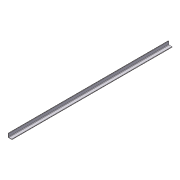
# Autodesk Inventor part: GE-12019-01
Saved by Autodesk Inventor 2012 (Build 160160000, 160)
## iProperties
Created: 2011-06-10
Part Number: GE-12019-01
Document SubType Name: Modeling
Designer: dfoster
Density: 2.71 g/cm^3
Material: Aluminum-6061
Mass: 4666.94 g
Surface Area: 5570.98 cm^2
Volume: 1722.12 cm^3
Description: Angle, Side
Title: Angle, Side
Author: dfoster
Autodesk Inventor part; units mm, degrees
ref_plane "YZ Plane" through (0, 0, 0) normal (1, 0, 0) x (0, 1, 0)
ref_plane "XZ Plane" through (0, 0, 0) normal (0, 1, 0) x (-1, 0, 0)
ref_plane "XY Plane" through (0, 0, 0) normal (0, 0, 1) x (1, 0, 0)
sketch "Sketch1" plane through (0, 0, 0) normal (0, 0, 1) x (1, 0, 0)
  line L0 (0, 0) -> (0, 50.8)
  line L1 (0, 50.8) -> (3.175, 50.8)
  line L2 (50.8, 0) -> (0, 0)
  line L3 (6.35, 47.625) -> (6.35, 12.7)
  line L4 (12.7, 6.35) -> (47.625, 6.35)
  line L5 (50.8, 3.175) -> (50.8, 0)
  arc A0 (6.35, 12.7) -> (12.7, 6.35) centre (12.7, 12.7) ccw
  arc A1 (50.8, 3.175) -> (47.625, 6.35) centre (47.625, 3.175) ccw
  arc A2 (6.35, 47.625) -> (3.175, 50.8) centre (3.175, 47.625) ccw
  point P0 (6.35, 50.8)
  dimension "d0" = 50.8
  dimension "d7" = 6.35
  dimension "d14" = 6.35
  dimension "d15" = 3.175
  constraints: 12 end point, 7 perpendicular, 6 point on circle, 6 tangent, 3 centre point, 2 point on line, 1 equal radius, 1 vertical
  measures "d0" distance of L0.start L0.end
  measures "d7" distance between parallel lines of L0 L3
  measures "d14" radius of A0
  measures "d15" radius of A1
extrude "Extrusion1" add sketch "Sketch1" along normal blind 2133.6
body "Solid1"
